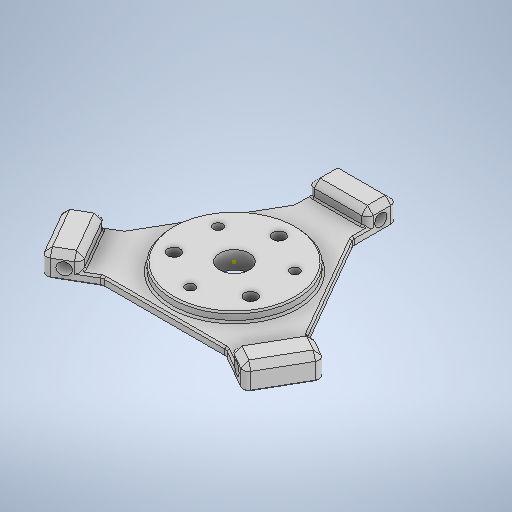
# Autodesk Inventor part: Base_E
Saved by Autodesk Inventor 2025 (Build 290162000, 162)
## iProperties
Created: 2026-06-13
Part Number: Base_E
Material: Generic
Document SubType Name: Sheet Metal
Designer: MSI
Density: 1 g/cm^3
Sheet Metal Rule: Default_mm
Appearance: Default
Author: MSI
Autodesk Inventor part; units mm, degrees
ref_plane "YZ Plane" through (0, 0, 0) normal (1, 0, 0) x (0, 1, 0)
ref_plane "XZ Plane" through (0, 0, 0) normal (0, 1, 0) x (-1, 0, 0)
ref_plane "XY Plane" through (0, 0, 0) normal (0, 0, 1) x (1, 0, 0)
sketch "Sketch1" plane through (0, 0, 0) normal (0, 1, 0) x (-1, 0, 0)
  line L0 (0, -40) -> (0, 0)
  line L1 (34.641, 20) -> (0, 0)
  line L2 (-34.641, 20) -> (0, 0)
  line L3 (-10, -43) -> (-10, -37)
  line L4 (-8, -35) -> (8, -35)
  line L5 (10, -37) -> (10, -43)
  arc A0 (10, -37) -> (8, -35) centre (8, -37) ccw
  arc A1 (8, -45) -> (10, -43) centre (8, -43) ccw
  arc A2 (-10, -43) -> (-8, -45) centre (-8, -43) ccw
  arc A3 (-8, -35) -> (-10, -37) centre (-8, -37) ccw
  line L6 (8, -45) -> (-8, -45)
  arc A4 (27.0429, 27.1603) -> (26.3109, 24.4282) centre (28.0429, 25.4282) ccw
  arc A5 (34.3109, 10.5718) -> (37.0429, 9.8397) centre (36.0429, 11.5718) ccw
  line L7 (42.2391, 12.8397) -> (37.0429, 9.8397)
  line L8 (27.0429, 27.1603) -> (32.2391, 30.1603)
  arc A6 (34.9711, 29.4282) -> (32.2391, 30.1603) centre (33.2391, 28.4282) ccw
  arc A7 (42.2391, 12.8397) -> (42.9711, 15.5718) centre (41.2391, 14.5718) ccw
  line L9 (34.9711, 29.4282) -> (42.9711, 15.5718)
  line L10 (34.3109, 10.5718) -> (26.3109, 24.4282)
  arc A8 (-37.0429, 9.8397) -> (-34.3109, 10.5718) centre (-36.0429, 11.5718) ccw
  arc A9 (-26.3109, 24.4282) -> (-27.0429, 27.1603) centre (-28.0429, 25.4282) ccw
  line L11 (-32.2391, 30.1603) -> (-27.0429, 27.1603)
  line L12 (-37.0429, 9.8397) -> (-42.2391, 12.8397)
  arc A10 (-42.9711, 15.5718) -> (-42.2391, 12.8397) centre (-41.2391, 14.5718) ccw
  arc A11 (-32.2391, 30.1603) -> (-34.9711, 29.4282) centre (-33.2391, 28.4282) ccw
  line L13 (-42.9711, 15.5718) -> (-34.9711, 29.4282)
  line L14 (-26.3109, 24.4282) -> (-34.3109, 10.5718)
  line L15 (29.641, 28.6603) -> (21.4449, 23.9282)
  line L16 (39.641, 11.3397) -> (31.4449, 6.6077)
  line L17 (-39.641, 11.3397) -> (-31.4449, 6.6077)
  line L18 (-29.641, 28.6603) -> (-21.4449, 23.9282)
  line L19 (10, -40) -> (10, -30.5359)
  line L20 (-10, -40) -> (-10, -30.5359)
  line L21 (20.4449, 23.6603) -> (-20.4449, 23.6603)
  line L22 (-30.7128, 5.8756) -> (-10.2679, -29.5359)
  line L23 (10.2679, -29.5359) -> (30.7128, 5.8756)
  arc A12 (20.4449, 23.6603) -> (21.4449, 23.9282) centre (20.4449, 25.6603) ccw
  arc A13 (31.4449, 6.6077) -> (30.7128, 5.8756) centre (32.4449, 4.8756) ccw
  arc A14 (10.2679, -29.5359) -> (10, -30.5359) centre (12, -30.5359) ccw
  arc A15 (-30.7128, 5.8756) -> (-31.4449, 6.6077) centre (-32.4449, 4.8756) ccw
  arc A16 (-21.4449, 23.9282) -> (-20.4449, 23.6603) centre (-20.4449, 25.6603) ccw
  arc A17 (-10, -30.5359) -> (-10.2679, -29.5359) centre (-12, -30.5359) ccw
  arc A18 (-28.541, 28.0252) -> (-38.541, 10.7047) centre (0, 0) ccw
  arc A19 (-10, -38.7298) -> (10, -38.7298) centre (0, 0) ccw
  arc A20 (38.541, 10.7047) -> (28.541, 28.0252) centre (0, 0) ccw
  circle A21 centre (0, 0) radius 21
  circle A22 centre (0, 0) radius 5
  circle A23 centre (0, -15) radius 2.1
  circle A24 centre (12.9904, 7.5) radius 2.1
  circle A25 centre (-12.9904, 7.5) radius 2.1
  circle A26 centre (-12.9904, -7.5) radius 1.6
  circle A27 centre (12.9904, -7.5) radius 1.6
  circle A28 centre (0, 15) radius 1.6
  point P0 (-10, -45)
  point P1 (43.9711, 13.8397)
  point P2 (-33.9711, 31.1603)
  point P3 (20.9808, 23.6603)
  point P4 (30.9808, 6.3397)
  point P5 (-30.9808, 6.3397)
  point P6 (-20.9808, 23.6603)
  point P7 (10, -30)
  point P8 (-10, -30)
  point P9 (-37.0429, 9.8397)
  point P10 (-27.0429, 27.1603)
  dimension "d3" = 360
  dimension "d14" = 360
  dimension "d20" = 360
  dimension "d22" = 2
  dimension "d23" = 42
  dimension "d29" = 360
  dimension "d41" = 360
  constraints: 48 end point, 42 point on circle, 29 centre point, 21 point on line, 18 tangent, 8 equal radius, 6 coincident, 2 horizontal, 2 midpoint, 1 perpendicular, 111 other
  measures "d22" radius of A12
  measures "d23" diameter of A21
extrude "Extrusion1" add sketch "Sketch1" along normal blind 3 contours L4 A3 L20 A17 L22 A15 L17 A8 L14 L2 A21 L0 | L0 A21 L1 L10 A5 L16 A13 L23 A14 L19 A0 L4 | L2 L14 A9 L18 A16 L21 A12 L15 A4 L10 L1 A21
extrude "Extrusion2" add sketch "Sketch1" along normal blind 6 contours A21 L2 A25 A22 L0 A23 | L0 A23 A22 L1 A24 A21 | A21 L1 A24 A22 L2 A25
extrude "Extrusion3" add sketch "Sketch1" along normal blind 8 contours A19 L3 A3 L4 L0 | A19 L5 A1 L6 A2 L3 | L0 L4 A0 L5 A19 | L14 A8 L12 A18 L2 | L2 A18 L11 A9 L14 | A18 L12 A10 L13 A11 L11 | L10 A4 L8 A20 L1 | L1 A20 L7 A5 L10 | A20 L8 A6 L9 A7 L7
chamfer "Chamfer1" distance 2 angle 45 24 edges at (33.7567, 8, 30.3601) (38.9711, 8, 22.5) (43.1709, 8, 14.0542) (39.641, 8, 11.3397) (35.5253, 8, 9.6399) (30.3109, 8, 17.5) (26.1111, 8, 25.9458) (29.641, 8, 28.6603) (10, 8, -40) (9.4142, 8, -44.4142) (0, 8, -45) (-9.4142, 8, -44.4142) (-10, 8, -40) (-9.4142, 8, -35.5858) (0, 8, -35) (9.4142, 8, -35.5858) (-29.641, 8, 28.6603) (-26.1111, 8, 25.9458) (-30.3109, 8, 17.5) (-35.5253, 8, 9.6399) (-39.641, 8, 11.3397) (-43.1709, 8, 14.0542) (-38.9711, 8, 22.5) (-33.7567, 8, 30.3601)
sketch "Sketch2" plane through (10, 0, -30.5359) normal (1, 0, 0) x (0, 0, -1)
  line L0 (6, 3.5) -> (9, 3.5)
  circle A0 centre (9, 3.5) radius 2.05
  line L1 (6.4641, 6) -> (12.4641, 6) projected
  point P0 (-30.5359, 0)
  dimension "d52" = 3
  dimension "d53" = 4.1
  dimension "d68" = 2.5
  constraints: 2 end point, 1 centre point, 1 coincident, 1 horizontal
  measures "d52" distance of L0.start L0.end
  measures "d53" diameter of A0
  measures "d68" distance from line of L1 L0.end
extrude "Extrusion4" cut sketch "Sketch2" against normal blind 20
pattern_circular "Circular Pattern1" count 3 over 360 about axis through (0, 0, 0) along (0, 1, 0) of "Extrusion4"
chamfer "Chamfer2" distance 0.6 angle 45 16 edges at (21, 3, 0) (20.4904, 3, -11.8301) (10.0681, 3, -30.0183) (10, 3, -33.7679) (31.0307, 3, 6.2899) (34.2439, 3, 8.2237) (-20.4904, 3, -11.8301) (-31.0307, 3, 6.2899) (-34.2439, 3, 8.2237) (-10.0681, 3, -30.0183) (-10, 3, -33.7679) (0, 3, 23.6603) (20.9625, 3, 23.7284) (24.2439, 3, 25.5442) (-20.9625, 3, 23.7284) (-24.2439, 3, 25.5442)
chamfer "Chamfer3" distance 0.5 angle 45 1 edges at (21, 6, 0)
chamfer "Chamfer4" distance 0.5 angle 45 24 edges at (20.4904, 0, -11.8301) (10.0681, 0, -30.0183) (10, 0, -36.7679) (9.4142, 0, -44.4142) (0, 0, -45) (-9.4142, 0, -44.4142) (-10, 0, -36.7679) (-10.0681, 0, -30.0183) (-20.4904, 0, -11.8301) (-31.0307, 0, 6.2899) (-36.842, 0, 9.7237) (-43.1709, 0, 14.0542) (-38.9711, 0, 22.5) (-33.7567, 0, 30.3601) (-26.842, 0, 27.0442) (-20.9625, 0, 23.7284) (0, 0, 23.6603) (20.9625, 0, 23.7284) (26.842, 0, 27.0442) (33.7567, 0, 30.3601) (38.9711, 0, 22.5) (43.1709, 0, 14.0542) (36.842, 0, 9.7237) (31.0307, 0, 6.2899)
chamfer "Chamfer5" distance 0.5 angle 45 9 edges at (30.3109, 3, 17.5) (34.8175, 3, 9.9912) (26.0614, 3, 25.1572) (-30.3109, 3, 17.5) (-26.0614, 3, 25.1572) (-34.8175, 3, 9.9912) (0, 3, -35) (-8.7561, 3, -35.1484) (8.7561, 3, -35.1484)
sketch "Sketch3" plane through (0, 6, 0) normal (0, 1, 0) x (1, 0, 0)
  point P0 (0, 0)
equation "\"BendRadius\" = Thickness"
equation "\"BendReliefWidth\" = Thickness"
equation "\"BendReliefDepth\" = 0.5 * Thickness"
equation "\"CornerReliefSize\" = 4 * Thickness"
equation "\"MinimumRemnant\" = 2 * Thickness"
equation "\"TransitionRadius\" = BendRadius"
equation "\"JacobiRadiusSize\" = BendRadius"
equation "\"GapSize\" = Thickness"
equation "\"Thickness\" = 0.5"
body "Solid1"
